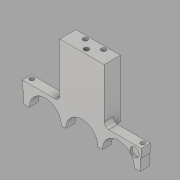
# Autodesk Inventor part: Tube Holder with camera attachment
Saved by Autodesk Inventor 2017 (Build 210142000, 142)
## iProperties
Created: 2016-12-06
Part Number: Tube Holder with camera attachment
Material: Aluminum 6061-AHC
Document SubType Name: Modeling
Designer: qupec
Density: 2.7 g/cm^3
Appearance: Aluminum - Dark
Mass: 40.9656 g
Surface Area: 72.5902 cm^2
Volume: 15.1725 cm^3
Author: qupec
Autodesk Inventor part; units mm, degrees
ref_plane "YZ Plane" through (0, 0, 0) normal (1, 0, 0) x (0, 1, 0)
ref_plane "XZ Plane" through (0, 0, 0) normal (0, 1, 0) x (-1, 0, 0)
ref_plane "XY Plane" through (0, 0, 0) normal (0, 0, 1) x (1, 0, 0)
sketch "Sketch1" plane through (0, 0, 0) normal (0, 0, 1) x (1, 0, 0)
  line L0 (-41.783, 14.2875) -> (41.783, 14.2875)
  line L1 (41.783, 14.2875) -> (41.783, -14.2875)
  line L2 (41.783, -14.2875) -> (-41.783, -14.2875)
  line L3 (-41.783, -14.2875) -> (-41.783, 14.2875)
  point P0 (0, 0)
  dimension "d0" = 83.566
  dimension "d1" = 41.783
  dimension "d2" = 14.2875
  dimension "d3" = 28.575
  constraints: 8 end point, 2 parallel, 1 horizontal, 1 perpendicular
  measures "d0" distance of L0.start L0.end
  measures "d1" distance from line of point (0, 0) L3
  measures "d2" distance from line of point (0, 0) L2
  measures "d3" distance of L2.end L0.start
extrude "Extrusion1" add sketch "Sketch1" along normal mid plane 6.35
sketch "Sketch2" plane through (0, 0, 3.175) normal (0, 0, 1) x (1, 0, 0)
  circle A0 centre (-25.781, 0) radius 11.303
  circle A1 centre (0, 0) radius 11.303
  line L0 (41.783, -14.2875) -> (41.783, 14.2875) projected
  circle A2 centre (25.781, 0) radius 11.303
  line L1 (-41.783, 14.2875) -> (-41.783, -14.2875) projected
  line L2 (-41.783, 0) -> (41.783, 0) construction
  line L3 (41.783, 14.2875) -> (-41.783, 14.2875) projected
  point P0 (0, 0)
  dimension "d6" = 22.606
  dimension "d9" = 22.606
  dimension "d11" = 22.606
  dimension "d14" = 25.781
  dimension "d21" = 83.566
  dimension "d22" = 25.781
  dimension "d50" = 0
  dimension "d150" = 3.175
  constraints: 3 centre point, 3 midpoint, 2 end point, 1 point on line
  measures "d6" diameter of A0
  measures "d9" diameter of A1
  measures "d11" diameter of A2
  measures "d14" distance of A1.centre A0.centre
  measures "d21" distance of L0.end L1.start
  measures "d22" distance of A2.centre A1.centre
  measures "d50" distance of point (0, 0) A1.centre
sketch "Sketch4" plane through (-41.783, -14.2875, -3.175) normal (-1, 0, 0) x (0, 0, 1)
  line L0 (0, 0) -> (0, 28.575) projected
  line L1 (6.35, 28.575) -> (6.35, 0) projected
  line L2 (0, 22.6695) -> (6.35, 22.6695)
  line L3 (6.35, 22.6695) -> (6.35, 5.9055)
  line L4 (6.35, 5.9055) -> (0, 5.9055)
  line L5 (0, 5.9055) -> (0, 22.6695)
  point P0 (3.175, 14.2875)
  dimension "d30" = 8.382
  dimension "d31" = 16.764
  constraints: 8 end point, 2 parallel, 1 horizontal, 1 perpendicular, 1 point on line, 2 other
  measures "d30" distance from line of point (3.175, 14.287) L4
  measures "d31" distance between parallel lines of L4 L2
extrude "Extrusion3" cut sketch "Sketch4" against normal blind 0.635
mirror "Mirror1" about plane through (0, 0, 0) normal (1, 0, 0) of "Extrusion3"
sketch "Sketch5" plane through (0, 0, 3.175) normal (0, 0, 1) x (1, 0, 0)
  circle A0 centre (0, 9.7155) radius 3.175 construction
  line L0 (41.783, 14.2875) -> (-41.783, 14.2875) projected
  line L1 (-17.7594, 20.454) -> (41.148, 0) construction
  line L2 (41.148, 8.382) -> (41.148, -8.382) projected
  circle A1 centre (2.8334, 17.8757) radius 3.175 construction
  circle A2 centre (36.576, 1.5875) radius 3.175 construction
  circle A3 centre (-36.576, 26.9875) radius 3.175 construction
  line L3 (-41.148, 8.382) -> (-41.148, -8.382) projected
  circle A4 centre (37.211, 9.7155) radius 3.175
  circle A5 centre (-37.211, -9.7155) radius 3.175
  line L4 (41.783, 8.382) -> (41.783, 14.2875) projected
  line L5 (-41.783, -14.2875) -> (41.783, -14.2875) projected
  line L6 (-41.783, -14.2875) -> (-41.783, -8.382) projected
  point P0 (0, 0)
  dimension "d34" = 6.35
  dimension "d35" = 4.572
  dimension "d53" = 6.35
  dimension "d54" = 6.35
  dimension "d55" = 4.572
  dimension "d56" = 4.572
  dimension "d57" = 12.7
  dimension "d58" = 6.35
  dimension "d59" = 6.35
  dimension "d60" = 4.572
  dimension "d61" = 4.572
  dimension "d62" = 4.572
  dimension "d63" = 4.572
  constraints: 6 centre point, 2 end point, 2 point on line, 1 midpoint, 1 symmetric about line, 1 other
  measures "d34" diameter of A0
  measures "d35" distance from line of L0 A0.centre
  measures "d53" diameter of A2
  measures "d54" diameter of A3
  measures "d55" distance from line of L2 A2.centre
  measures "d56" distance from line of L3 A3.centre
  measures "d57" distance from line of L0 A2.centre
  measures "d58" diameter of A4
  measures "d59" diameter of A5
  measures "d60" distance from line of L4 A4.centre
  measures "d61" distance from line of L0 A4.centre
  measures "d62" distance from line of L5 A5.centre
  measures "d63" distance from line of L6 A5.centre
extrude "Extrusion4" cut sketch "Sketch5" against normal blind 1.27
sketch "Sketch7" plane through (-41.783, -14.2875, 3.175) normal (0, -1, 0) x (1, 0, 0)
  line L0 (27.813, -14.605) -> (55.753, -14.605)
  line L1 (55.753, -14.605) -> (55.753, 8.255)
  line L2 (55.753, 8.255) -> (27.813, 8.255)
  line L3 (27.813, 8.255) -> (27.813, -14.605)
  point P0 (41.783, -3.175)
  dimension "d39" = 27.94
  dimension "d40" = 22.86
  dimension "d41" = 11.43
  dimension "d42" = 13.97
  constraints: 8 end point, 2 parallel, 1 horizontal, 1 perpendicular
  measures "d39" distance of L0.start L0.end
  measures "d40" distance of L2.end L0.start
  measures "d41" distance from line of point (41.783, -3.175) L0
  measures "d42" distance from line of point (41.783, -3.175) L1
extrude "Extrusion5" [suppressed]
sketch "Sketch8" plane through (0, 0, -3.175) normal (0, 0, -1) x (-1, 0, 0)
  line L0 (-41.783, 14.2875) -> (41.783, 14.2875) projected
  line L1 (15.6718, 14.2875) -> (-15.6718, 14.2875)
  line L2 (-15.6718, 14.2875) -> (-15.6718, 52.3875)
  line L3 (-15.6718, 52.3875) -> (15.6718, 52.3875)
  line L4 (15.6718, 52.3875) -> (15.6718, 14.2875)
  point P0 (0, 0)
  dimension "d45" = 31.3436
  dimension "d46" = 38.1
  dimension "d47" = 15.6718
  constraints: 8 end point, 2 parallel, 1 horizontal, 1 perpendicular, 1 point on line
  measures "d45" distance between parallel lines of L2 L4
  measures "d46" distance between parallel lines of L0 L3
  measures "d47" distance from line of point (0, 0) L4
extrude "Extrusion6" add sketch "Sketch8" against normal up to surface (6.35 mm away)
extrude "Extrusion7" cut sketch "Sketch2" against normal blind 25.4
sketch "Sketch9" plane through (-15.6718, 52.3875, -3.175) normal (0, 1, 0) x (1, 0, 0)
  line L0 (-26.1112, -6.35) -> (57.4548, -6.35) projected
  line L1 (3.1718, -6.35) -> (28.1718, -6.35)
  line L2 (28.1718, -6.35) -> (28.1718, -3.175)
  line L3 (28.1718, -3.175) -> (3.1718, -3.175)
  line L4 (3.1718, -3.175) -> (3.1718, -6.35)
  point P0 (15.6718, -3.175)
  dimension "d64" = 3.175
  dimension "d65" = 25
  dimension "d66" = 12.5
  constraints: 8 end point, 2 parallel, 1 horizontal, 1 perpendicular, 1 point on line
  measures "d64" distance of L3.end L1.start
  measures "d65" distance of L2.end L3.end
  measures "d66" distance from line of point (15.672, -3.175) L4
extrude "Extrusion8" [suppressed]
sketch "Sketch13" plane through (0, 0, 3.175) normal (0, 0, 1) x (1, 0, 0)
  line L0 (-41.783, -8.382) -> (-41.783, -14.2875) projected
  line L1 (-41.783, -14.2875) -> (41.783, -14.2875) projected
  line L2 (41.783, -14.2875) -> (41.783, -8.382) projected
  line L3 (41.783, -8.382) -> (41.148, -8.382) projected
  line L4 (-41.148, -8.382) -> (-41.783, -8.382) projected
  line L5 (-41.148, -8.382) -> (-41.148, 0)
  line L6 (-41.148, 8.382) -> (-41.148, -8.382) projected
  line L7 (-41.148, 0) -> (41.148, 0)
  line L8 (41.148, 8.382) -> (41.148, -8.382) projected
  line L9 (41.148, 0) -> (41.148, -8.382)
  point P0 (0, 0)
  constraints: 6 end point, 2 midpoint, 1 collinear
extrude "Extrusion11" cut sketch "Sketch13" against normal through all
sketch "Sketch14" plane through (37.084, 0, 3.175) normal (0, -1, 0) x (1, 0, 0)
  line L0 (4.064, -6.35) -> (0, -6.35) projected
  line L1 (4.064, 0) -> (4.064, -6.35) projected
  line L2 (0, 0) -> (4.064, 0) projected
  line L3 (0, -6.35) -> (0, 0) projected
  line L4 (-3.048, -1.27) -> (3.302, -1.27) projected
  circle A0 centre (2.032, -3.81) radius 1.5494
  point P0 (-37.084, -3.175)
  dimension "d84" = 3.0988
  dimension "d85" = 6.35
  dimension "d86" = 5.08
  dimension "d87" = 4.064
  dimension "d88" = 2.032
  dimension "d89" = 2.54
  constraints: 1 centre point
  measures "d84" diameter of A0
  measures "d85" distance of L4.start L4.end
  measures "d86" distance between parallel lines of L0 L4
  measures "d87" distance between parallel lines of L1 L3
  measures "d88" distance from line of L1 A0.centre
  measures "d89" distance from line of L4 A0.centre
extrude "Extrusion12" cut sketch "Sketch14" against normal through all contours A0
mirror "Mirror3" about plane through (0, 0, 0) normal (1, 0, 0) of "Extrusion12"
thread "Thread3" size "5-40 UNC" class "2B" standard "ANSI Unified Screw Threads" length 12.7 offset 6.35
thread "Thread4" size "5-40 UNC" class "2B" standard "ANSI Unified Screw Threads" length 12.7 offset 6.35
sketch "Sketch15" plane through (-15.6718, 52.3875, -3.175) normal (0, 1, 0) x (1, 0, 0)
  line L0 (0, -6.35) -> (0, 0) projected
  line L1 (0, 0) -> (3.175, 0)
  line L2 (3.175, 0) -> (3.175, 5.08)
  line L3 (3.175, 5.08) -> (0, 5.08)
  line L4 (0, 5.08) -> (0, 0)
  line L5 (31.3436, 0) -> (0, 0) construction
  line L6 (11.5062, 0) -> (19.8374, 0)
  line L7 (31.3436, 0) -> (28.1686, 0)
  line L8 (28.1686, 0) -> (28.1686, 5.08)
  line L9 (28.1686, 5.08) -> (31.3436, 5.08)
  line L10 (31.3436, 5.08) -> (31.3436, 0)
  line L11 (31.3436, 0) -> (31.3436, -6.35) projected
  line L12 (4.3688, 0) -> (26.9748, 0) projected
  line L13 (19.8374, 0) -> (28.1686, 0)
  point P0 (15.6718, -3.175)
  point P1 (19.8374, 5.08)
  point P2 (3.175, 0.8467)
  dimension "d96" = 5.08
  dimension "d102" = 31.3436
  dimension "d105" = 3.175
  dimension "d106" = 3.175
  dimension "d120" = 5.08
  constraints: 20 end point, 4 parallel, 3 horizontal, 3 point on line, 2 perpendicular, 1 collinear
  measures "d96" distance of L3.end L0.end
  measures "d102" distance between parallel lines of L11 L0
  measures "d105" distance of L2.end L3.end
  measures "d106" distance of L8.end L9.end
  measures "d120" distance between parallel lines of L5 L9
sketch "Sketch16" plane through (-15.6718, 52.3875, 3.175) normal (0, 1, 0) x (1, 0, 0)
  line L0 (31.3436, 6.35) -> (0, 6.35) projected
  arc A0 (8.3312, 6.35) -> (11.5062, 6.35) centre (9.9187, 6.35) ccw
  line L1 (11.5062, 10.5833) -> (11.5062, 6.35) projected
  line L2 (8.3312, 6.35) -> (8.3312, 10.5833) projected
  line L3 (4.3688, 6.35) -> (26.9748, 6.35) projected
  arc A1 (19.8374, 6.35) -> (23.0124, 6.35) centre (21.4249, 6.35) ccw
  line L4 (23.0124, 10.5833) -> (23.0124, 6.35) projected
  line L5 (19.8374, 6.35) -> (19.8374, 10.5833) projected
  point P0 (15.6718, 3.175)
  constraints: 4 point on circle, 4 point on line, 4 tangent, 2 centre point, 2 end point
extrude "Extrusion15" [suppressed]
fillet "Fillet3" [suppressed]
fillet "Fillet4" [suppressed]
fillet "Fillet5" radius 3.175 2 edges at (15.6718, 14.2875, 0) (-15.6718, 14.2875, 0)
extrude "Extrusion16" add sketch "Sketch15" against normal blind 40.64
sketch "Sketch17" plane through (-15.6718, 52.3875, 3.175) normal (0, 1, 0) x (1, 0, 0)
  line L0 (28.1686, 6.35) -> (28.1686, 11.43) projected
  line L1 (3.175, 11.43) -> (3.175, 6.35) projected
  line L2 (28.1686, 11.43) -> (3.175, 11.43)
  line L3 (3.175, 11.43) -> (3.175, 6.35)
  line L4 (3.175, 6.35) -> (28.1686, 6.35)
  line L5 (28.1686, 6.35) -> (28.1686, 11.43)
  point P0 (15.6718, 3.175)
  constraints: 8 end point, 2 parallel, 1 horizontal, 1 perpendicular
extrude "Extrusion17" add sketch "Sketch17" against normal blind 3.175
fillet "Fillet6" radius 3.175 2 edges at (-12.4968, 49.2125, -5.715) (12.4968, 49.2125, -5.715)
sketch "Sketch18" plane through (-15.6718, 52.3875, 3.175) normal (0, 1, 0) x (1, 0, 0)
  circle A0 centre (9.2964, 8.89) radius 1.6764
  circle A1 centre (22.0472, 8.89) radius 1.6764
  line L0 (31.3436, 11.43) -> (0, 11.43) projected
  line L1 (6.35, 6.35) -> (24.9936, 6.35) projected
  line L2 (6.35, 11.43) -> (6.35, 6.35) projected
  line L3 (24.9936, 6.35) -> (24.9936, 11.43) projected
  line L4 (7.62, 8.89) -> (23.7236, 8.89) construction
  point P0 (15.6718, 3.175)
  point P1 (23.7236, 8.89)
  dimension "d126" = 3.3528
  dimension "d127" = 3.3528
  dimension "d128" = 5.08
  dimension "d129" = 2.54
  dimension "d130" = 2.54
  dimension "d132" = 1.27
  dimension "d134" = 1.27
  constraints: 2 end point, 2 point on circle, 1 centre point, 1 horizontal alignment, 2 other
  measures "d127" diameter of A1
  measures "d128" distance between parallel lines of L0 L1
  measures "d129" distance from line of point (9.296, 8.89) L1
  measures "d130" distance from line of L1 A1.centre
  measures "d132" distance from line of L2 L4.start
  measures "d134" distance from line of L3 L4.end
extrude "Extrusion18" cut sketch "Sketch18" against normal through all contours A0 | A1
sketch "Sketch19" plane through (-15.6718, 52.3875, 3.175) normal (0, 1, 0) x (1, 0, 0)
  line L0 (6.35, 6.35) -> (24.9936, 6.35) projected
  line L1 (0, 0) -> (31.3436, 0) projected
  circle A0 centre (15.6718, 3.175) radius 1.6764
  dimension "d137" = 3.3528
  constraints: 1 centre point, 1 coincident
  measures "d137" diameter of A0
extrude "Extrusion19" cut sketch "Sketch19" against normal blind 12.7
thread "Thread5" size "6-32 UNC" class "2B" standard "ANSI Unified Screw Threads" full length
sketch "Sketch20" plane through (-15.6718, 52.3875, 3.175) normal (0, 1, 0) x (1, 0, 0)
  circle A0 centre (9.2964, 8.89) radius 1.6764 projected
  circle A1 centre (15.6718, 3.175) radius 1.6764 projected
  circle A2 centre (9.2964, 8.89) radius 1.6764 projected
  circle A3 centre (22.0472, 8.89) radius 1.6764 projected
  line L0 (0, 0) -> (31.3436, 0) projected
  line L1 (31.3436, 11.43) -> (31.3436, 0) projected
  line L2 (31.3436, 11.43) -> (0, 11.43) projected
  line L3 (0, 11.43) -> (0, 0) projected
  dimension "d142" = 2.54
  dimension "d143" = 9.2964
  dimension "d144" = 8.255
  measures "d142" distance from line of L2 A0.centre
  measures "d143" distance from line of L3 A0.centre
  measures "d144" distance from line of point (15.672, 3.175) L2
equation "\"d1\" = 0.5 * d0"
equation "\"d2\" = 0.5 * d3"
equation "\"d9\" = d7"
equation "\"d11\" = d9"
equation "\"d22\" = d14"
equation "\"d30\" = 0.5 * d31"
equation "\"d41\" = 0.5 * d40"
equation "\"d42\" = 0.5 * d39"
equation "\"d47\" = 0.5 * d45"
equation "\"d66\" = 0.5 * d65"
equation "\"d88\" = 0.5 * d87"
equation "\"d89\" = 0.5 * d86"
equation "\"d106\" = d105"
equation "\"d120\" = d96"
equation "\"d127\" = d126"
equation "\"d129\" = 0.5 * d128"
equation "\"d130\" = 0.5 * d128"
equation "\"d134\" = d132"
equation "\"d7\" = d6"
body "Solid1"
